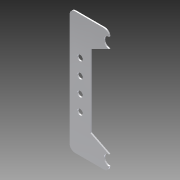
# Autodesk Inventor part: V5 Shooter Guide Rail Support Plate
Saved by Autodesk Inventor 2014 SP1 (Build 180222100, 222)
## iProperties
Created: 2012-02-13
Part Number: V5 Shooter Guide Rail Support Plate
Material: Aluminum-6061
Document SubType Name: Modeling
Designer: Moses
Density: 2.71 g/cm^3
Mass: 19.8474 g
Surface Area: 100.393 cm^2
Volume: 7.32375 cm^3
Appearance: Aluminum - Polished
Author: Moses
Autodesk Inventor part; units mm, degrees
ref_plane "YZ Plane" through (0, 0, 0) normal (1, 0, 0) x (0, 1, 0)
ref_plane "XZ Plane" through (0, 0, 0) normal (0, 1, 0) x (-1, 0, 0)
ref_plane "XY Plane" through (0, 0, 0) normal (0, 0, 1) x (1, 0, 0)
sketch "Sketch1" plane through (0, 0, 0) normal (0, 0, 1) x (1, 0, 0)
  circle A0 centre (31.75, 28.575) radius 3.3782 projected
  circle A1 centre (31.75, 9.525) radius 3.3782 projected
  circle A2 centre (31.75, -9.525) radius 3.3782 projected
  circle A3 centre (31.75, -28.575) radius 3.3782 projected
  circle A4 centre (67.1293, 62.0712) radius 6.35 construction
  circle A5 centre (67.1293, -62.0713) radius 6.35 construction
  line L0 (19.05, 74.7712) -> (19.05, -74.7713)
  line L1 (19.05, -74.7713) -> (67.1293, -74.7713)
  line L2 (67.1293, -74.7713) -> (67.1293, -68.4213)
  line L3 (19.05, 74.7712) -> (67.1293, 74.7712)
  line L4 (67.1293, 74.7712) -> (67.1293, 68.4212)
  line L5 (67.1293, 62.0712) -> (67.1293, 55.7212) construction
  line L6 (67.1293, -55.7213) -> (67.1293, -62.0713) construction
  line L7 (44.45, 44.45) -> (44.45, -44.45)
  line L8 (44.45, -44.45) -> (67.1293, -55.7213)
  line L9 (44.45, 44.45) -> (67.1293, 55.7212)
  arc A6 (67.1293, 68.4212) -> (67.1293, 55.7212) centre (67.1293, 62.0712) ccw
  line L10 (67.1293, 68.4212) -> (67.1293, 62.0712) construction
  arc A7 (67.1293, -55.7213) -> (67.1293, -68.4213) centre (67.1293, -62.0713) ccw
  line L11 (67.1293, -62.0713) -> (67.1293, -68.4213) construction
  point P0 (0, 0)
  dimension "d0" = 88.9
  dimension "d2" = 12.7
  dimension "d3" = 12.7
  dimension "d4" = 12.7
  dimension "d5" = 12.7
  constraints: 24 end point, 8 point on circle, 3 collinear, 3 parallel, 3 perpendicular, 2 centre point, 2 coincident, 1 equal length, 1 vertical
  measures "d0" distance of L7.start L7.end
  measures "d2" distance of L3.end L5.start
  measures "d3" distance from line of A0.centre L0
  measures "d4" distance from line of L7 A0.centre
  measures "d5" distance of L1.end L6.end
extrude "Extrusion1" add sketch "Sketch1" along normal blind 1.5875
fillet "Fillet1" radius 6.35 4 edges at (67.1293, 74.7712, 0.7937) (67.1293, -74.7713, 0.7937) (19.05, -74.7713, 0.7937) (19.05, 74.7712, 0.7937)
equation "\"d4\" = d3"
equation "\"d5\" = d2"
body "Solid1"
